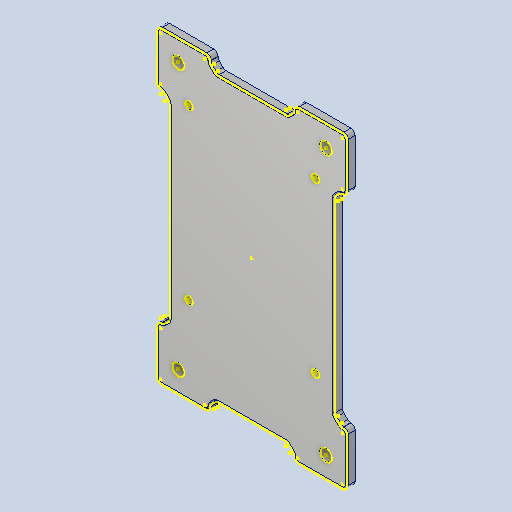
# Autodesk Inventor part: EllipseFix
Saved by Autodesk Inventor 2022 (Build 260153000, 153)
## iProperties
Created: 2019-04-14
Part Number: EllipseFix
Material: Generic
Document SubType Name: Modeling
Designer: CASE-SMALL2
Density: 1 g/cm^3
Appearance: Default
Author: CASE-SMALL2
Autodesk Inventor part; units mm, degrees
ref_plane "YZ Plane" through (0, 0, 0) normal (1, 0, 0) x (0, 1, 0)
ref_plane "XZ Plane" through (0, 0, 0) normal (0, 1, 0) x (-1, 0, 0)
ref_plane "XY Plane" through (0, 0, 0) normal (0, 0, 1) x (1, 0, 0)
sketch "Sketch1" plane through (0, 0, 0) normal (0, 0, 1) x (1, 0, 0)
  line L0 (-45, -73) -> (45, -73)
  line L1 (45, -73) -> (45, 73)
  line L2 (45, 73) -> (-45, 73)
  line L3 (-45, 73) -> (-45, -73)
  line L4 (-45, -73) -> (45, 73) construction
  line L5 (45, -73) -> (-45, 73) construction
  point P0 (0, 0)
  dimension "d0" = 90
  dimension "d1" = 146
  constraints: 12 end point, 2 midpoint, 2 parallel, 1 horizontal, 1 perpendicular
  measures "d0" distance of L1.end L2.end
  measures "d1" distance of L0.end L1.end
extrude "Extrusion1" add sketch "Sketch1" along normal blind 4
sketch "Sketch2" plane through (0, 0, 4) normal (0, 0, 1) x (1, 0, 0)
  circle A0 centre (-35, -63) radius 2.75
  line L0 (-45, -73) -> (45, -73) projected
  line L1 (-45, 73) -> (-45, -73) projected
  line L2 (-77.5799, 0) -> (77.5799, 0) projected
  line L3 (0, 102.7799) -> (0, -102.7799) projected
  circle A1 centre (-35, 63) radius 2.75
  circle A2 centre (35, -63) radius 2.75
  circle A3 centre (35, 63) radius 2.75
  point P0 (0, 0)
  dimension "d4" = 5.5
  dimension "d5" = 10
  dimension "d6" = 10
  constraints: 4 centre point, 3 symmetric about line, 3 other
  measures "d4" diameter of A0
  measures "d5" distance from line of L0 A0.centre
  measures "d6" distance from line of L1 A0.centre
extrude "Extrusion2" cut sketch "Sketch2" against normal up to surface (4 mm away) contours A0 | A1 | A2 | A3
sketch "Sketch3" plane through (0, 0, 0) normal (0, 0, -1) x (-1, 0, 0)
  circle A0 centre (-30, -32) radius 1.75
  circle A1 centre (-30, 48) radius 1.75
  circle A2 centre (30, -32) radius 1.75
  circle A3 centre (30, 48) radius 1.75
  line L0 (0, -102.7799) -> (0, 102.7799) projected
  line L1 (-45, 73) -> (45, 73) projected
  point P0 (0, 0)
  dimension "d9" = 3.5
  dimension "d10" = 3.5
  dimension "d11" = 3.5
  dimension "d12" = 3.5
  dimension "d13" = 80
  dimension "d15" = 80
  dimension "d16" = 30
  dimension "d17" = 30
  dimension "d18" = 30
  dimension "d19" = 30
  dimension "d20" = 25
  dimension "d21" = 25
  constraints: 4 centre point
  measures "d9" diameter of A0
  measures "d10" diameter of A1
  measures "d11" diameter of A2
  measures "d12" diameter of A3
  measures "d13" distance of A1.centre A0.centre
  measures "d15" distance of A3.centre A2.centre
  measures "d16" distance from line of L0 A0.centre
  measures "d17" distance from line of L0 A2.centre
  measures "d18" distance from line of L0 A3.centre
  measures "d19" distance from line of L0 A1.centre
  measures "d20" distance from line of L1 A1.centre
  measures "d21" distance from line of L1 A3.centre
extrude "Extrusion3" cut sketch "Sketch3" against normal up to surface (4 mm away)
sketch "Sketch4" plane through (0, 0, 4) normal (0, 0, 1) x (1, 0, 0)
  line L0 (-45, 73) -> (-45, -73) construction
  line L1 (-45, 48) -> (-42, 48)
  line L2 (-42, 48) -> (-39, 45)
  line L3 (-39, 45) -> (-39, -45)
  line L4 (-39, -45) -> (-42, -48)
  line L5 (-42, -48) -> (-45, -48)
  line L6 (-45, -48) -> (-45, 48)
  line L7 (-45, -73) -> (45, -73) construction
  line L8 (45, 73) -> (-45, 73) construction
  line L9 (-20, -73) -> (-20, -70)
  line L10 (-20, -70) -> (-17, -67)
  line L11 (-17, -67) -> (17, -67)
  line L12 (17, -67) -> (20, -70)
  line L13 (20, -70) -> (20, -73)
  line L14 (45, -73) -> (45, 73) projected
  line L15 (0, -102.7799) -> (0, 102.7799) construction
  line L16 (-77.5799, 0) -> (77.5799, 0) construction
  line L17 (45, 73) -> (45, -73) construction
  line L18 (45, 48) -> (42, 48)
  line L19 (42, 48) -> (39, 45)
  line L20 (39, 45) -> (39, -45)
  line L21 (39, -45) -> (42, -48)
  line L22 (42, -48) -> (45, -48)
  line L23 (45, -48) -> (45, 48)
  line L24 (-20, -73) -> (20, -73)
  line L25 (-20, 73) -> (-20, 70)
  line L26 (-20, 70) -> (-17, 67)
  line L27 (-17, 67) -> (17, 67)
  line L28 (17, 67) -> (20, 70)
  line L29 (20, 70) -> (20, 73)
  line L30 (-20, 73) -> (20, 73)
  point P0 (0, 0)
  dimension "d24" = 25
  dimension "d25" = 6
  dimension "d26" = 135
  dimension "d27" = 25
  dimension "d28" = 135
  dimension "d29" = 3
  dimension "d30" = 3
  dimension "d31" = 6
  dimension "d32" = 3
  dimension "d33" = 3
  dimension "d34" = 135
  dimension "d35" = 25
  dimension "d36" = 25
  constraints: 50 end point, 12 symmetric about line, 6 perpendicular, 6 point on line, 1 collinear, 1 parallel, 1 vertical
  measures "d24" distance between parallel lines of L8 L1
  measures "d25" distance between parallel lines of L0 L3
  measures "d26" angle of L1 L2
  measures "d27" distance between parallel lines of L7 L5
  measures "d28" angle of L3 L4
  measures "d29" distance of L4.end L5.end
  measures "d30" distance of L1.start L1.end
  measures "d31" distance between parallel lines of L7 L11
  measures "d32" distance of L12.end L13.end
  measures "d33" distance of L9.start L9.end
  measures "d34" angle of L11 L10
  measures "d35" distance between parallel lines of L0 L9
  measures "d36" distance between parallel lines of L14 L13
extrude "Extrusion4" cut sketch "Sketch4" against normal up to surface (4 mm away)
fillet "Fillet1" radius 2 28 edges at (-45, 73, 2) (-20, 73, 2) (-45, 48, 2) (-39, 45, 2) (-42, 48, 2) (-39, -45, 2) (-42, -48, 2) (-45, -48, 2) (-45, -73, 2) (-20, -73, 2) (-20, -70, 2) (-17, -67, 2) (17, -67, 2) (20, -70, 2) (20, -73, 2) (45, -73, 2) (39, -45, 2) (42, -48, 2) (45, -48, 2) (39, 45, 2) (42, 48, 2) (45, 48, 2) (45, 73, 2) (20, 73, 2) (20, 70, 2) (17, 67, 2) (-17, 67, 2) (-20, 70, 2)
sketch "Sketch5" plane through (0, 0, 4) normal (0, 0, 1) x (1, 0, 0)
  circle A0 centre (-30, -32) radius 1.75 projected
  circle A1 centre (-30, 48) radius 1.75 projected
  circle A2 centre (30, 48) radius 1.75 projected
  circle A3 centre (30, -32) radius 1.75 projected
  circle A4 centre (35, -63) radius 2.75 projected
  circle A5 centre (35, 63) radius 2.75 projected
  circle A6 centre (-35, 63) radius 2.75 projected
  circle A7 centre (-35, -63) radius 2.75 projected
  arc A8 (22, 73) -> (20, 71) centre (22, 71) ccw projected
  line L0 (20, 71) -> (20, 70.8284) projected
  arc A9 (19.4142, 69.4142) -> (20, 70.8284) centre (18, 70.8284) ccw projected
  line L1 (19.4142, 69.4142) -> (17.5858, 67.5858) projected
  arc A10 (16.1716, 67) -> (17.5858, 67.5858) centre (16.1716, 69) ccw projected
  line L2 (16.1716, 67) -> (-16.1716, 67) projected
  arc A11 (-17.5858, 67.5858) -> (-16.1716, 67) centre (-16.1716, 69) ccw projected
  line L3 (-17.5858, 67.5858) -> (-19.4142, 69.4142) projected
  arc A12 (-20, 70.8284) -> (-19.4142, 69.4142) centre (-18, 70.8284) ccw projected
  line L4 (-20, 70.8284) -> (-20, 71) projected
  arc A13 (-20, 71) -> (-22, 73) centre (-22, 71) ccw projected
  line L5 (-22, 73) -> (-43, 73) projected
  arc A14 (-43, 73) -> (-45, 71) centre (-43, 71) ccw projected
  line L6 (-45, 71) -> (-45, 50) projected
  arc A15 (-45, 50) -> (-43, 48) centre (-43, 50) ccw projected
  line L7 (-43, 48) -> (-42.8284, 48) projected
  arc A16 (-41.4142, 47.4142) -> (-42.8284, 48) centre (-42.8284, 46) ccw projected
  line L8 (-41.4142, 47.4142) -> (-39.5858, 45.5858) projected
  arc A17 (-39, 44.1716) -> (-39.5858, 45.5858) centre (-41, 44.1716) ccw projected
  line L9 (-39, 44.1716) -> (-39, -44.1716) projected
  arc A18 (-39.5858, -45.5858) -> (-39, -44.1716) centre (-41, -44.1716) ccw projected
  line L10 (-39.5858, -45.5858) -> (-41.4142, -47.4142) projected
  arc A19 (-42.8284, -48) -> (-41.4142, -47.4142) centre (-42.8284, -46) ccw projected
  line L11 (-42.8284, -48) -> (-43, -48) projected
  arc A20 (-43, -48) -> (-45, -50) centre (-43, -50) ccw projected
  line L12 (-45, -50) -> (-45, -71) projected
  arc A21 (-45, -71) -> (-43, -73) centre (-43, -71) ccw projected
  line L13 (-43, -73) -> (-22, -73) projected
  arc A22 (-22, -73) -> (-20, -71) centre (-22, -71) ccw projected
  line L14 (-20, -71) -> (-20, -70.8284) projected
  arc A23 (-19.4142, -69.4142) -> (-20, -70.8284) centre (-18, -70.8284) ccw projected
  line L15 (-19.4142, -69.4142) -> (-17.5858, -67.5858) projected
  arc A24 (-16.1716, -67) -> (-17.5858, -67.5858) centre (-16.1716, -69) ccw projected
  line L16 (-16.1716, -67) -> (16.1716, -67) projected
  arc A25 (17.5858, -67.5858) -> (16.1716, -67) centre (16.1716, -69) ccw projected
  line L17 (17.5858, -67.5858) -> (19.4142, -69.4142) projected
  arc A26 (20, -70.8284) -> (19.4142, -69.4142) centre (18, -70.8284) ccw projected
  line L18 (20, -70.8284) -> (20, -71) projected
  arc A27 (20, -71) -> (22, -73) centre (22, -71) ccw projected
  line L19 (22, -73) -> (43, -73) projected
  arc A28 (43, -73) -> (45, -71) centre (43, -71) ccw projected
  line L20 (45, -71) -> (45, -50) projected
  arc A29 (45, -50) -> (43, -48) centre (43, -50) ccw projected
  line L21 (43, -48) -> (42.8284, -48) projected
  arc A30 (41.4142, -47.4142) -> (42.8284, -48) centre (42.8284, -46) ccw projected
  line L22 (41.4142, -47.4142) -> (39.5858, -45.5858) projected
  arc A31 (39, -44.1716) -> (39.5858, -45.5858) centre (41, -44.1716) ccw projected
  line L23 (39, -44.1716) -> (39, 44.1716) projected
  arc A32 (39.5858, 45.5858) -> (39, 44.1716) centre (41, 44.1716) ccw projected
  line L24 (39.5858, 45.5858) -> (41.4142, 47.4142) projected
  arc A33 (42.8284, 48) -> (41.4142, 47.4142) centre (42.8284, 46) ccw projected
  line L25 (42.8284, 48) -> (43, 48) projected
  arc A34 (43, 48) -> (45, 50) centre (43, 50) ccw projected
  line L26 (45, 50) -> (45, 71) projected
  arc A35 (45, 71) -> (43, 73) centre (43, 71) ccw projected
  line L27 (43, 73) -> (22, 73) projected
  point P0 (0, 0)
chamfer "Chamfer1" distance 0.75 angle 45 56 edges at (0, -67, 4) (16.9369, -67.1522, 4) (18.5, -68.5, 4) (19.8478, -70.0631, 4) (20, -70.9142, 4) (20.5858, -72.4142, 4) (32.5, -73, 4) (44.4142, -72.4142, 4) (45, -60.5, 4) (44.4142, -48.5858, 4) (42.9142, -48, 4) (42.0631, -47.8478, 4) (40.5, -46.5, 4) (39.1522, -44.9369, 4) (39, 0, 4) (39.1522, 44.9369, 4) (40.5, 46.5, 4) (42.0631, 47.8478, 4) (42.9142, 48, 4) (44.4142, 48.5858, 4) (45, 60.5, 4) (44.4142, 72.4142, 4) (32.5, 73, 4) (20.5858, 72.4142, 4) (20, 70.9142, 4) (19.8478, 70.0631, 4) (18.5, 68.5, 4) (16.9369, 67.1522, 4) (0, 67, 4) (-16.9369, 67.1522, 4) (-18.5, 68.5, 4) (-19.8478, 70.0631, 4) (-20, 70.9142, 4) (-20.5858, 72.4142, 4) (-32.5, 73, 4) (-44.4142, 72.4142, 4) (-45, 60.5, 4) (-44.4142, 48.5858, 4) (-42.9142, 48, 4) (-42.0631, 47.8478, 4) (-40.5, 46.5, 4) (-39.1522, 44.9369, 4) (-39, 0, 4) (-39.1522, -44.9369, 4) (-40.5, -46.5, 4) (-42.0631, -47.8478, 4) (-42.9142, -48, 4) (-44.4142, -48.5858, 4) (-45, -60.5, 4) (-44.4142, -72.4142, 4) (-32.5, -73, 4) (-20.5858, -72.4142, 4) (-20, -70.9142, 4) (-19.8478, -70.0631, 4) (-18.5, -68.5, 4) (-16.9369, -67.1522, 4)
equation "\"d10\" = d9"
equation "\"d11\" = d9"
equation "\"d12\" = d9"
equation "\"d15\" = d13"
equation "\"d17\" = d16"
equation "\"d18\" = d16"
equation "\"d19\" = d16"
equation "\"d21\" = d20"
equation "\"d27\" = d24"
equation "\"d30\" = d29"
equation "\"d36\" = d35"
body "Solid1"
